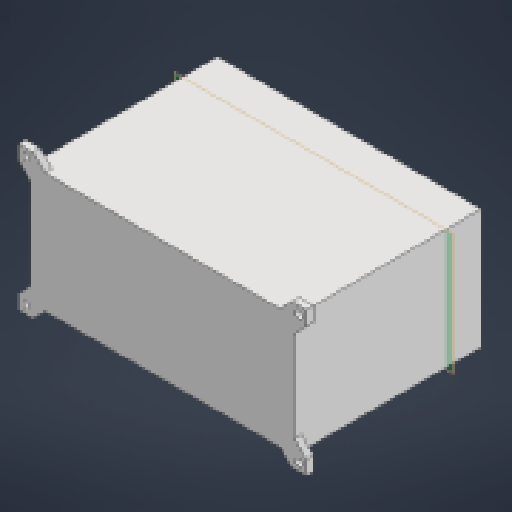
# Autodesk Inventor part: lvl202x01_toggle_body
Saved by Autodesk Inventor 2024 (Build 280153000, 153)
## iProperties
Created: 2026-04-07
Part Number: lvl202x01_toggle_body
Material: Generic
Document SubType Name: Modeling
Designer: schar
Density: 1 g/cm^3
Appearance: Default
Author: schar
Autodesk Inventor part; units mm, degrees
ref_plane "YZ Plane" through (0, 0, 0) normal (1, 0, 0) x (0, 1, 0)
ref_plane "XZ Plane" through (0, 0, 0) normal (0, 1, 0) x (-1, 0, 0)
ref_plane "XY Plane" through (0, 0, 0) normal (0, 0, 1) x (1, 0, 0)
sketch "Sketch1" plane through (0, 0, 0) normal (0, 0, 1) x (1, 0, 0)
  line L0 (-55, 25) -> (55, 25)
  line L1 (55, 25) -> (55, -25)
  line L2 (55, -25) -> (-55, -25)
  line L3 (-55, -25) -> (-55, 25)
  line L4 (-55, 25) -> (55, -25) construction
  line L5 (55, 25) -> (-55, -25) construction
  line L6 (-55, 25) -> (-49, 25)
  line L7 (-60, 30) -> (60, 30)
  line L8 (60, 30) -> (60, -30)
  line L9 (60, -30) -> (-60, -30)
  line L10 (-60, -30) -> (-60, 30)
  line L11 (-60, 30) -> (60, -30) construction
  line L12 (60, 30) -> (-60, -30) construction
  line L13 (-60, 30) -> (-54, 30)
  line L14 (-54, 30) -> (-49, 25)
  line L15 (-55, 25) -> (-55, 19)
  line L16 (-55, 19) -> (-60, 24)
  circle A0 centre (-56.768, 26.768) radius 1.5 projected
  circle A1 centre (-56.768, 26.768) radius 1.5
  line L17 (55, 25) -> (49, 25)
  line L18 (60, 30) -> (54, 30)
  line L19 (54, 30) -> (49, 25)
  line L20 (55, 25) -> (55, 19)
  line L21 (60, 30) -> (60, 24)
  line L22 (60, 24) -> (55, 19)
  line L23 (55, -25) -> (49, -25)
  line L24 (55, -25) -> (55, -19)
  line L25 (60, -30) -> (60, -24)
  line L26 (60, -30) -> (54, -30)
  line L27 (54, -30) -> (49, -25)
  line L28 (55, -19) -> (60, -24)
  line L29 (-55, -25) -> (-49, -25)
  line L30 (-55, -25) -> (-55, -19)
  line L31 (-60, -30) -> (-60, -24)
  line L32 (-60, -24) -> (-55, -19)
  line L33 (-49, -25) -> (-54, -30)
  circle A2 centre (56.768, 26.768) radius 1.5 projected
  circle A3 centre (56.768, -26.768) radius 1.5 projected
  circle A4 centre (-56.768, -26.768) radius 1.5 projected
  point P0 (0, 0)
  dimension "d0" = 110
  dimension "d1" = 50
  dimension "d2" = 6
  dimension "d3" = 120
  dimension "d4" = 60
  dimension "d5" = 6
  dimension "d6" = 6
  dimension "d7" = 6
  dimension "d8" = 6
  dimension "d9" = 6
  dimension "d10" = 6
  dimension "d11" = 6
  dimension "d12" = 6
  dimension "d13" = 6
  dimension "d14" = 6
  dimension "d15" = 6
  dimension "d16" = 6
  constraints: 68 end point, 16 point on line, 6 parallel, 4 midpoint, 2 horizontal, 2 perpendicular, 1 centre point, 1 coincident, 1 concentric
  measures "d0" distance of L1.end L2.end
  measures "d1" distance of L0.end L1.end
  measures "d2" distance of L0.start L6.end
  measures "d3" distance of L8.end L9.end
  measures "d4" distance of L7.end L8.end
  measures "d5" distance of L7.start L13.end
  measures "d6" distance of L0.end L17.end
  measures "d7" distance of L7.end L18.end
  measures "d8" distance of L0.end L20.end
  measures "d9" distance of L7.end L21.end
  measures "d10" distance of L1.end L23.end
  measures "d11" distance of L1.end L24.end
  measures "d12" distance of L8.end L25.end
  measures "d13" distance of L8.end L26.end
  measures "d14" distance of L2.end L29.end
  measures "d15" distance of L2.end L30.end
  measures "d16" distance of L9.end L31.end
extrude "Extrusion1" add sketch "Sketch1" along normal blind 3 contours L3 L16 L10 L7 L14 L0 | L0 L1 L2 L3 | L19 L7 L8 L22 L1 L0 | L3 L2 L33 L9 L10 L32 | L28 L8 L9 L27 L2 L1
sketch "Sketch2" plane through (0, 0, 0) normal (0, 0, -1) x (-1, 0, 0)
  line L0 (-55, 25) -> (55, 25)
  line L1 (55, 25) -> (55, -25)
  line L2 (55, -25) -> (-55, -25)
  line L3 (-55, -25) -> (-55, 25)
  line L4 (-55, 25) -> (55, -25) construction
  line L5 (55, 25) -> (-55, -25) construction
  line L6 (-55, 25) -> (55, 25)
  line L7 (55, 25) -> (55, -25)
  line L8 (55, -25) -> (-55, -25)
  line L9 (-55, -25) -> (-55, 25)
  line L10 (-55, 25) -> (55, -25) construction
  line L11 (55, 25) -> (-55, -25) construction
  line L12 (-53.2, 23.2) -> (53.2, 23.2)
  line L13 (53.2, 23.2) -> (53.2, -23.2)
  line L14 (53.2, -23.2) -> (-53.2, -23.2)
  line L15 (-53.2, -23.2) -> (-53.2, 23.2)
  line L16 (-53.2, 23.2) -> (53.2, -23.2) construction
  line L17 (53.2, 23.2) -> (-53.2, -23.2) construction
  point P0 (0, 0)
  point P1 (-55, -23)
  point P2 (55, -23)
  point P3 (55, 23)
  point P4 (-55, 23)
  point P5 (-53.2, 25)
  point P6 (-53.2, -25)
  point P7 (53.2, -25)
  point P8 (53.2, 25)
  dimension "d19" = 110
  dimension "d20" = 50
  dimension "d21" = 106.4
  dimension "d22" = 46.4
  constraints: 36 end point, 6 midpoint, 6 parallel, 3 horizontal, 3 perpendicular
  measures "d19" distance of L1.end L2.end
  measures "d20" distance of L0.end L1.end
  measures "d21" distance of L13.end L14.end
  measures "d22" distance of L12.end L13.end
extrude "Extrusion2" add sketch "Sketch2" along normal blind 75
ref_plane "Work Plane1" through (0, 0, -60) normal (0, 0, -1) x (-1, 0, 0)
sketch "Sketch8" plane through (0, 0, 0) normal (0, 0, -1) x (-1, 0, 0)
  line L0 (-53.2, 23.2) -> (-53.2, -23.2) projected
  line L1 (-53.2, 0) -> (-36.2, 0)
  line L2 (53.2, 23.2) -> (53.2, -23.2) projected
  line L3 (53.2, 0) -> (36.2, 0)
  circle A0 centre (-36.2, 0) radius 6
  circle A1 centre (36.2, 0) radius 6
  circle A2 centre (0, 0) radius 6
  dimension "d55" = 17
  dimension "d56" = 17
  dimension "d57" = 12
  dimension "d58" = 12
  dimension "d59" = 12
  constraints: 4 end point, 3 centre point, 3 coincident, 2 horizontal, 2 midpoint
  measures "d55" distance of L1.start L1.end
  measures "d56" distance of L3.start L3.end
  measures "d57" diameter of A0
  measures "d58" diameter of A1
  measures "d59" diameter of A2
extrude "Extrusion7" cut sketch "Sketch8" against normal blind 75
fillet "Fillet1" radius 2 4 edges at (-60, 30, 1.5) (60, 30, 1.5) (60, -30, 1.5) (-60, -30, 1.5)
body "Solid1"
